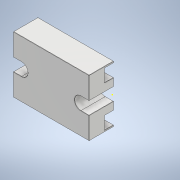
# Autodesk Inventor part: Solid State Rele SSR40DA
Saved by Autodesk Inventor 2020 (Build 240168000, 168)
## iProperties
Created: 2019-06-07
Part Number: Solid State Rele SSR40DA
Material: Пластмасса, непрозрачная, белая
Document SubType Name: Modeling
Designer: Boss
Mass: 41.5321 g
Surface Area: 108.516 cm^2
Volume: 43.6261 cm^3
Density: 0.952 g/cm^3
Appearance: Гладкий — белый
Длинна: 60,000 мм
Ширина: 45,000 мм
Author: Boss
Autodesk Inventor part; units mm, degrees
ref_plane "YZ Plane" through (0, 0, 0) normal (1, 0, 0) x (0, 1, 0)
ref_plane "XZ Plane" through (0, 0, 0) normal (0, 1, 0) x (-1, 0, 0)
ref_plane "XY Plane" through (0, 0, 0) normal (0, 0, 1) x (1, 0, 0)
sketch "Эскиз1" plane through (0, 0, 0) normal (0, 1, 0) x (-1, 0, 0)
  line L0 (0, 0) -> (80, 0) construction
  line L1 (0, 0) -> (0, -22.5)
  line L2 (0, -22.5) -> (60, -22.5)
  line L3 (60, -22.5) -> (60, 0)
  line L4 (0, 0) -> (0, 22.5)
  line L5 (0, 22.5) -> (60, 22.5)
  line L6 (60, 22.5) -> (60, 0)
  point P0 (40, 0)
  dimension "d0" = 80
  dimension "Высота" = 22.5
  dimension "Длинна" = 60
  constraints: 14 end point, 2 perpendicular, 2 symmetric about line, 1 horizontal alignment, 1 midpoint, 1 parallel, 1 point on line
  measures "d0" distance of L0.start L0.end
  measures "Высота" distance of L0.start L1.end
  measures "Длинна" distance of L1.end L2.end
extrude "Выдавливание1" add sketch "Эскиз1" along normal blind 19.5
sketch "Эскиз2" plane through (0, 19.5, 0) normal (0, 1, 0) x (1, 0, 0)
  line L0 (-60, 22.5) -> (-60, -22.5) projected
  line L1 (0, -22.5) -> (0, 22.5) projected
  line L2 (-60, 0) -> (0, 0) construction
  arc A0 (-6.5, 5) -> (-6.5, -5) centre (-6.5, 0) ccw
  line L3 (-6.5, 5) -> (0, 5)
  line L4 (-6.5, -5) -> (0, -5)
  line L5 (-30, 0) -> (-30, 10) construction
  arc A1 (-53.5, -5) -> (-53.5, 5) centre (-53.5, 0) ccw
  line L6 (-53.5, 5) -> (-60, 5)
  line L7 (-53.5, -5) -> (-60, -5)
  line L8 (-14, 11.25) -> (0, 11.25)
  line L9 (0, 11.25) -> (0, 21.25)
  line L10 (0, 21.25) -> (-14, 21.25)
  line L11 (-14, 21.25) -> (-14, 11.25)
  line L12 (-14, -11.25) -> (0, -11.25)
  line L13 (0, -11.25) -> (0, -21.25)
  line L14 (0, -21.25) -> (-14, -21.25)
  line L15 (-14, -21.25) -> (-14, -11.25)
  line L16 (0, -5) -> (0, 5)
  line L17 (-60, -5) -> (-60, 5)
  line L18 (-60, 11.75) -> (-48, 11.75)
  line L19 (-48, 11.75) -> (-48, 20.75)
  line L20 (-48, 20.75) -> (-60, 20.75)
  line L21 (-60, 20.75) -> (-60, 11.75)
  line L22 (-60, -11.75) -> (-48, -11.75)
  line L23 (-48, -11.75) -> (-48, -20.75)
  line L24 (-48, -20.75) -> (-60, -20.75)
  line L25 (-60, -20.75) -> (-60, -11.75)
  line L26 (-16.5, 21) -> (-45.2, 21)
  line L27 (-45.2, -21) -> (-16.5, -21)
  line L28 (-16.5, -21) -> (-16.5, 21)
  line L29 (-45.2, 21) -> (-45.2, -21)
  point P0 (-48, 16.25)
  point P1 (-14, 16.25)
  point P2 (-48, -16.25)
  point P3 (-7, -16.25)
  point P4 (-7, -11.25)
  point P5 (-14, -16.25)
  point P6 (-7, 16.25)
  point P7 (-54, -16.25)
  point P8 (-54, -11.75)
  point P9 (-48, -16.25)
  point P10 (-54, 16.25)
  dimension "d5" = 5
  dimension "d6" = 6.5
  dimension "d7" = 10
  dimension "d8" = 14
  dimension "d9" = 10
  dimension "d10" = 22.5
  dimension "d15" = 12
  dimension "d16" = 9
  dimension "d18" = 1.5
  dimension "d41" = 2.5
  dimension "d42" = 28.7
  dimension "d43" = 16
  constraints: 56 end point, 17 symmetric about line, 10 perpendicular, 8 midpoint, 4 point on circle, 3 horizontal alignment, 2 centre point, 2 collinear, 2 parallel, 2 point on line, 2 tangent, 2 vertical alignment, 1 other
  measures "d5" radius of A0
  measures "d6" distance from line of A0.centre L1
  measures "d7" distance of L5.start L5.end
  measures "d8" distance of L10.end L9.end
  measures "d9" distance of L9.end L8.end
  measures "d10" diameter of L8.end L2
  measures "d15" distance of L20.end L19.end
  measures "d16" distance of L19.end L18.end
  measures "d18" distance from line of L0.end L27
  measures "d41" distance between parallel lines of L15 L28
  measures "d42" distance of L26.start L26.end
  measures "d43" distance between parallel lines of L26 L3
extrude "Выдавливание2" cut sketch "Эскиз2" against normal blind 19.5 contours L6 A1 L7 L0 | L4 A0 L3 L1
extrude "Выдавливание3" cut sketch "Эскиз2" against normal blind 7 contours L20 L19 L18 L0 | L22 L23 L24 L0 | L14 L15 L12 L1 | L8 L11 L10 L1
extrude "Выдавливание4" cut sketch "Эскиз2" against normal blind 1 contours L28 L27 L29 L26
fillet "Сопряжение1" radius 0.2 64 edges at (0, 0, 13.75) (0, 9.75, 5) (0, 19.5, 8.125) (0, 16, 11.25) (0, 12.5, 16.25) (0, 16, 21.25) (0, 19.5, 21.875) (0, 9.75, 22.5) (-30, 0, 22.5) (-60, 0, 13.75) (-56.75, 0, 5) (-48.5, 0, 0) (-56.75, 0, -5) (-60, 0, -13.75) (-30, 0, -22.5) (0, 0, -13.75) (-3.25, 0, -5) (-11.5, 0, 0) (-3.25, 0, 5) (-3.25, 19.5, 5) (-60, 19.5, 21.625) (-54, 19.5, 20.75) (-30, 19.5, 22.5) (-48, 19.5, 16.25) (-54, 19.5, 11.75) (-7, 19.5, 21.25) (-60, 19.5, 8.375) (-14, 19.5, 16.25) (-56.75, 19.5, 5) (-7, 19.5, 11.25) (-48.5, 19.5, 0) (-56.75, 19.5, -5) (-60, 19.5, -8.375) (-11.5, 19.5, 0) (-54, 19.5, -11.75) (-3.25, 19.5, -5) (-48, 19.5, -16.25) (0, 19.5, -8.125) (-54, 19.5, -20.75) (-7, 19.5, -11.25) (-60, 19.5, -21.625) (-14, 19.5, -16.25) (-30, 19.5, -22.5) (-7, 19.5, -21.25) (0, 19.5, -21.875) (-16.5, 19.5, 0) (-30.85, 19.5, -21) (-45.2, 19.5, 0) (-30.85, 19.5, 21) (-60, 9.75, 22.5) (-60, 16, 20.75) (-60, 12.5, 16.25) (-60, 16, 11.75) (-60, 9.75, 5) (-60, 9.75, -5) (-60, 16, -11.75) (-60, 12.5, -16.25) (-60, 16, -20.75) (-60, 9.75, -22.5) (0, 9.75, -22.5) (0, 16, -21.25) (0, 12.5, -16.25) (0, 16, -11.25) (0, 9.75, -5)
hole "Отверстие1" at (-7, 19.5, 16.25) at (-7, 19.5, -16.25) at (-54, 19.5, 16.25) at (-54, 19.5, -16.25) direction (0, -1, 0) diameter 4 depth 12 tip angle 118
sketch "Эскиз3" plane through (0, 18.5, 0) normal (0, 1, 0) x (1, 0, 0)
  line L0 (-45.1182, -21) -> (-45.1182, 20.9992) construction
  line L1 (-45.1182, 20.9992) -> (-16.5, 20.9992) construction
  line L2 (-16.5, 20.9992) -> (-16.5, -21) construction
  line L3 (-16.5, -21) -> (-45.1182, -21) construction
  point P0 (0, 0)
  constraints: 2 other
thread "Резьба1" size "M4x0.7" class "6H" standard "ANSI Metric M Profile" full length
thread "Резьба2" size "M4x0.7" class "6H" standard "ANSI Metric M Profile" full length
thread "Резьба3" size "M4x0.7" class "6H" standard "ANSI Metric M Profile" full length
thread "Резьба4" size "M4x0.7" class "6H" standard "ANSI Metric M Profile" full length
equation "\"Ширина\" = 45"
